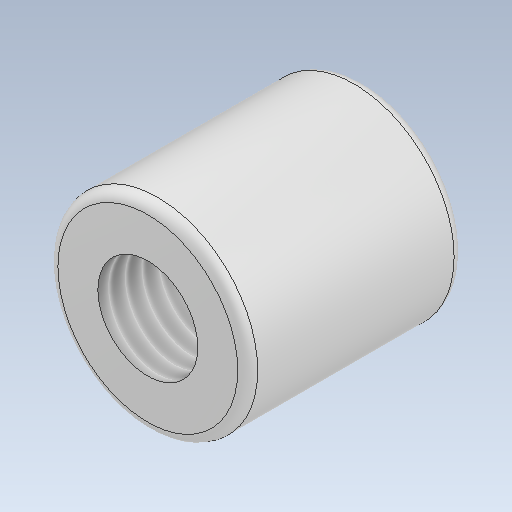
# Autodesk Inventor part: スペーサーM3L6.5黄銅
Saved by Autodesk Inventor 2020.2 (Build 242310000, 310)
## iProperties
Created: 2020-02-24
Part Number: スペーサーM3L6.5黄銅
Material: アルミニウム 2014-T4
Document SubType Name: Modeling
Designer: aoyam
Density: 2.8 g/cm^3
Appearance: サテン
Author: aoyam
Autodesk Inventor part; units mm, degrees
ref_plane "YZ Plane" through (0, 0, 0) normal (1, 0, 0) x (0, 1, 0)
ref_plane "XZ Plane" through (0, 0, 0) normal (0, 1, 0) x (-1, 0, 0)
ref_plane "XY Plane" through (0, 0, 0) normal (0, 0, 1) x (1, 0, 0)
sketch "スケッチ1" plane through (0, 0, 0) normal (0, 0, 1) x (1, 0, 0)
  circle A0 centre (0, 0) radius 1.5
  circle A1 centre (0, 0) radius 3
  dimension "d0" = 3
  dimension "d1" = 6
  constraints: 2 centre point, 2 coincident
  measures "d0" diameter of A0
  measures "d1" diameter of A1
extrude "押し出し1" add sketch "スケッチ1" along normal blind 6.5
fillet "フィレット1" radius 0.3 2 edges at (-3, 0, 6.5) (-3, 0, 0)
thread "ねじ1" size "M3x0.5" class "6H" standard "ANSI Metric M Profile" length 100
